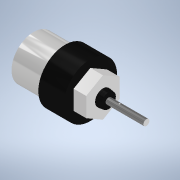
# Autodesk Inventor part: DC
Saved by Autodesk Inventor 2021 (Build 250183000, 183)
## iProperties
Created: 2021-07-14
Part Number: DC
Material: Aluminum 6061-AHC
Document SubType Name: Modeling
Designer: HP
Density: 2.7 g/cm^3
Appearance: Aluminum - Dark
Author: HP
Autodesk Inventor part; units mm, degrees
ref_plane "YZ Plane" through (0, 0, 0) normal (1, 0, 0) x (0, 1, 0)
ref_plane "XZ Plane" through (0, 0, 0) normal (0, 1, 0) x (-1, 0, 0)
ref_plane "XY Plane" through (0, 0, 0) normal (0, 0, 1) x (1, 0, 0)
sketch "Sketch1" plane through (0, 0, 0) normal (1, 0, 0) x (0, 1, 0)
  circle A0 centre (0, 0) radius 35
  dimension "d0" = 70
  constraints: 1 centre point, 1 coincident
  measures "d0" diameter of A0
extrude "Extrusion1" add sketch "Sketch1" along normal blind 50
sketch "Sketch2" plane through (50, 0, 0) normal (1, 0, 0) x (0, 0, -1)
  circle A0 centre (0, 0) radius 42.5
  dimension "d3" = 85
  constraints: 1 centre point, 1 coincident
  measures "d3" diameter of A0
extrude "Extrusion2" add sketch "Sketch2" along normal blind 40
sketch "Sketch3" plane through (90, 0, 0) normal (1, 0, 0) x (0, 0, -1)
  line L0 (0, 30.5873) -> (26.4894, 15.2937)
  line L1 (26.4894, 15.2937) -> (26.4894, -15.2937)
  line L2 (26.4894, -15.2937) -> (0, -30.5873)
  line L3 (0, -30.5873) -> (-26.4894, -15.2937)
  line L4 (-26.4894, -15.2937) -> (-26.4894, 15.2937)
  line L5 (-26.4894, 15.2937) -> (0, 30.5873)
  point P0 (0, 0)
  point P1 (0, 0)
  constraints: 12 end point, 1 coincident, 13 other
extrude "Extrusion3" add sketch "Sketch3" along normal blind 20
sketch "Sketch4" plane through (110, 0, 0) normal (1, 0, 0) x (0, 0, -1)
  circle A0 centre (0, 0) radius 12.5
  dimension "d8" = 25
  constraints: 1 centre point, 1 coincident
  measures "d8" diameter of A0
extrude "Extrusion4" add sketch "Sketch4" along normal blind 3
sketch "Sketch5" plane through (113, 0, 0) normal (1, 0, 0) x (0, 0, -1)
  circle A0 centre (0, 0) radius 12.0251
  constraints: 1 centre point, 1 coincident
extrude "Extrusion5" add sketch "Sketch5" along normal blind 3
sketch "Sketch6" plane through (116, 0, 0) normal (1, 0, 0) x (0, 0, -1)
  circle A0 centre (0, 0) radius 11.5831
  constraints: 1 centre point, 1 coincident
extrude "Extrusion6" add sketch "Sketch6" along normal blind 3
sketch "Sketch7" plane through (119, 0, 0) normal (1, 0, 0) x (0, 0, -1)
  circle A0 centre (0, 0) radius 4.75
  dimension "d16" = 9.5
  constraints: 1 centre point, 1 coincident
  measures "d16" diameter of A0
extrude "Extrusion7" add sketch "Sketch7" along normal blind 60
sketch "Sketch8" plane through (0, 0, 0) normal (0, 1, 0) x (-1, 0, 0)
  circle A0 centre (-136.5365, 0) radius 1.25
  point P0 (0, 0)
  dimension "d19" = 2.5
  constraints: 1 centre point
  measures "d19" diameter of A0
extrude "Extrusion8" cut sketch "Sketch8" along normal mid plane 20
body "Solid1"
